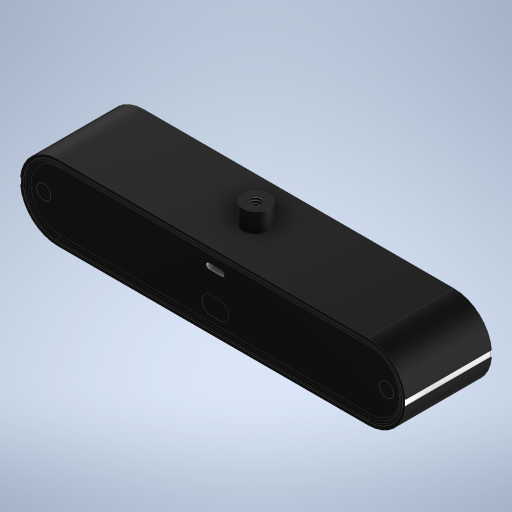
# Autodesk Inventor part: Astra
Saved by Autodesk Inventor 2024 (Build 280153000, 153)
## iProperties
Created: 2016-02-11
Part Number: Astra
Material: Generic
Document SubType Name: Modeling
Designer: John
Density: 1 g/cm^3
Appearance: Default
Author: John
Autodesk Inventor part; units mm, degrees
ref_plane "YZ Plane" through (0, 0, 0) normal (1, 0, 0) x (0, 1, 0)
ref_plane "XZ Plane" through (0, 0, 0) normal (0, 1, 0) x (-1, 0, 0)
sketch "Sketch1" plane through (0, 0, 0) normal (0, 1, 0) x (-1, 0, 0)
  line L0 (89.75, 0) -> (-89.75, 0) construction
  line L1 (72.2, 17.55) -> (-72.2, 17.55)
  line L2 (-72.2, -17.55) -> (72.2, -17.55)
  arc A0 (72.2, -17.55) -> (72.2, 17.55) centre (72.2, 0) ccw
  arc A1 (-72.2, 17.55) -> (-72.2, -17.55) centre (-72.2, 0) ccw
  point P0 (0, 0)
  point P1 (0, 0)
  dimension "d0" = 179.5
  dimension "d1" = 35.1
  constraints: 8 end point, 6 point on circle, 4 tangent, 2 centre point, 2 point on line, 1 coincident, 1 horizontal, 1 midpoint, 1 parallel
  measures "d0" distance of L0.start L0.end
  measures "d1" diameter of A1
extrude "Extrusion1" add sketch "Sketch1" along normal blind 40
sketch "Sketch2" plane through (0, 40, 0) normal (0, 1, 0) x (1, 0, 0)
  line L0 (-72.2, -17.55) -> (72.2, -17.55) projected
  arc A0 (72.2, -17.55) -> (72.2, 17.55) centre (72.2, 0) ccw projected
  line L1 (72.2, 17.55) -> (-72.2, 17.55) projected
  arc A1 (-72.2, 17.55) -> (-72.2, -17.55) centre (-72.2, 0) ccw projected
  line L2 (-72.2, 16.05) -> (72.2, 16.05)
  arc A2 (72.2, -16.05) -> (72.2, 16.05) centre (72.2, 0) ccw
  line L3 (72.2, -16.05) -> (-72.2, -16.05)
  arc A3 (-72.2, 16.05) -> (-72.2, -16.05) centre (-72.2, 0) ccw
  line L4 (-72.2, -14.55) -> (72.2, -14.55)
  arc A4 (72.2, -14.55) -> (72.2, 14.55) centre (72.2, 0) ccw
  line L5 (72.2, 14.55) -> (-72.2, 14.55)
  arc A5 (-72.2, 14.55) -> (-72.2, -14.55) centre (-72.2, 0) ccw
  point P0 (0, 0)
  dimension "d4" = 1.5
  dimension "d5" = 1.5
  constraints: 8 end point, 8 point on circle, 4 centre point, 6 other
  measures "d4" distance between parallel lines of L1 L2
  measures "d5" distance between parallel lines of L3 L4
extrude "Extrusion2" cut sketch "Sketch2" against normal blind 1 contours A5 L5 A4 L4
fillet "Fillet1" radius 1 8 edges at (-86.75, 39, 0) (0, 39, -14.55) (86.75, 39, 0) (0, 39, 14.55) (-86.75, 40, 0) (0, 40, -14.55) (86.75, 40, 0) (0, 40, 14.55)
sketch "Sketch3" plane through (0, 40, 0) normal (0, 1, 0) x (1, 0, 0)
  line L0 (-72.2, -17.55) -> (72.2, -17.55) projected
  arc A0 (72.2, -17.55) -> (72.2, 17.55) centre (72.2, 0) ccw projected
  line L1 (72.2, 17.55) -> (-72.2, 17.55) projected
  arc A1 (-72.2, 17.55) -> (-72.2, -17.55) centre (-72.2, 0) ccw projected
  arc A2 (-72.2, 15.2821) -> (-72.2, -15.2821) centre (-72.2, 0) ccw projected
  line L2 (72.2, 15.2821) -> (-72.2, 15.2821) projected
  arc A3 (72.2, -15.2821) -> (72.2, 15.2821) centre (72.2, 0) ccw projected
  line L3 (-72.2, -15.2821) -> (72.2, -15.2821) projected
  arc A4 (72.2, -15.95) -> (72.2, 15.95) centre (72.2, 0) ccw
  line L4 (72.2, 15.95) -> (-72.2, 15.95)
  arc A5 (-72.2, 15.95) -> (-72.2, -15.95) centre (-72.2, 0) ccw
  line L5 (-72.2, -15.95) -> (72.2, -15.95)
  line L6 (72.2, -16.05) -> (-72.2, -16.05)
  arc A6 (-72.2, 16.05) -> (-72.2, -16.05) centre (-72.2, 0) ccw
  line L7 (-72.2, 16.05) -> (72.2, 16.05)
  arc A7 (72.2, -16.05) -> (72.2, 16.05) centre (72.2, 0) ccw
  point P0 (0, 0)
  dimension "d12" = 1.5
  dimension "d13" = 0.1
  constraints: 8 end point, 8 point on circle, 4 centre point, 6 other
  measures "d12" distance between parallel lines of L0 L6
  measures "d13" distance between parallel lines of L5 L6
extrude "Extrusion3" cut sketch "Sketch3" against normal blind 1 contours L5 A5 L4 A4 | L6 A6 L7 A7
sketch "Sketch4" plane through (0, 0, 0) normal (0, -1, 0) x (1, 0, 0)
  line L0 (-72.2, 17.55) -> (72.2, 17.55) projected
  arc A0 (-72.2, 17.55) -> (-72.2, -17.55) centre (-72.2, 0) ccw projected
  line L1 (72.2, -17.55) -> (-72.2, -17.55) projected
  arc A1 (72.2, -17.55) -> (72.2, 17.55) centre (72.2, 0) ccw projected
  line L2 (72.2, 16.05) -> (-72.2, 16.05)
  arc A2 (-72.2, 16.05) -> (-72.2, -16.05) centre (-72.2, 0) ccw
  line L3 (-72.2, -16.05) -> (72.2, -16.05)
  arc A3 (72.2, -16.05) -> (72.2, 16.05) centre (72.2, 0) ccw
  line L4 (-72.2, 14.55) -> (72.2, 14.55)
  arc A4 (72.2, -14.55) -> (72.2, 14.55) centre (72.2, 0) ccw
  line L5 (72.2, -14.55) -> (-72.2, -14.55)
  arc A5 (-72.2, 14.55) -> (-72.2, -14.55) centre (-72.2, 0) ccw
  point P0 (0, 0)
  dimension "d14" = 1.5
  dimension "d15" = 1.5
  constraints: 8 end point, 8 point on circle, 4 centre point, 6 other
  measures "d14" distance between parallel lines of L0 L2
  measures "d15" distance between parallel lines of L2 L4
extrude "Extrusion4" cut sketch "Sketch4" against normal blind 1 contours L4 A4 L5 A5
fillet "Fillet2" radius 1 8 edges at (86.75, 1, 0) (0, 1, -14.55) (-86.75, 1, 0) (0, 1, 14.55) (86.75, 0, 0) (0, 0, -14.55) (-86.75, 0, 0) (0, 0, 14.55)
sketch "Sketch5" plane through (0, 0, 0) normal (0, -1, 0) x (1, 0, 0)
  line L0 (-72.2, 17.55) -> (72.2, 17.55) projected
  arc A0 (-72.2, 17.55) -> (-72.2, -17.55) centre (-72.2, 0) ccw projected
  line L1 (72.2, -17.55) -> (-72.2, -17.55) projected
  arc A1 (72.2, -17.55) -> (72.2, 17.55) centre (72.2, 0) ccw projected
  arc A2 (72.2, -15.2821) -> (72.2, 15.2821) centre (72.2, 0) ccw projected
  line L2 (-72.2, -15.2821) -> (72.2, -15.2821) projected
  arc A3 (-72.2, 15.2821) -> (-72.2, -15.2821) centre (-72.2, 0) ccw projected
  line L3 (72.2, 15.2821) -> (-72.2, 15.2821) projected
  line L4 (72.2, 16.05) -> (-72.2, 16.05)
  arc A4 (-72.2, 16.05) -> (-72.2, -16.05) centre (-72.2, 0) ccw
  line L5 (-72.2, -16.05) -> (72.2, -16.05)
  arc A5 (72.2, -16.05) -> (72.2, 16.05) centre (72.2, 0) ccw
  line L6 (-72.2, 16.15) -> (72.2, 16.15)
  arc A6 (72.2, -16.15) -> (72.2, 16.15) centre (72.2, 0) ccw
  line L7 (72.2, -16.15) -> (-72.2, -16.15)
  arc A7 (-72.2, 16.15) -> (-72.2, -16.15) centre (-72.2, 0) ccw
  point P0 (0, 0)
  dimension "d19" = 1.5
  dimension "d20" = 0.1
  constraints: 8 end point, 8 point on circle, 4 centre point, 6 other
  measures "d19" distance between parallel lines of L0 L4
  measures "d20" distance between parallel lines of L4 L6
extrude "Extrusion5" cut sketch "Sketch5" against normal blind 1 contours L6 A6 L7 A7
sketch "Sketch6" plane through (0, 39, 0) normal (0, 1, 0) x (1, 0, 0)
  line L0 (0, 0) -> (-60.5, 0) construction
  arc A0 (-61, 0.9108) -> (-61, -0.9108) centre (-60.5, 0) ccw construction
  arc A1 (-61.2406, 1.3491) -> (-61.2406, -1.3491) centre (-60.5, 0) ccw
  arc A2 (-60.7594, 0.4725) -> (-60.7594, -0.4725) centre (-60.5, 0) ccw
  arc A3 (-60.7594, 0.4725) -> (-61.2406, 1.3491) centre (-61, 0.9108) ccw
  arc A4 (-61.2406, -1.3491) -> (-60.7594, -0.4725) centre (-61, -0.9108) ccw
  line L1 (-60.5, 1) -> (-60.5, -1) construction
  dimension "d23" = 60.5
  dimension "d25" = 0.5
  dimension "d26" = 1
  dimension "d27" = 1
  dimension "d28" = 0
  constraints: 10 point on circle, 6 tangent, 5 centre point, 4 end point, 1 coincident, 1 horizontal, 1 vertical
  measures "d23" distance of L0.start L0.end
  measures "d25" radius of A3
  measures "d26" distance of L0.end L1.end
  measures "d27" distance of L0.end L1.start
  measures "d28" distance from line of L1 L0.end
extrude "mic" cut sketch "Sketch6" against normal blind 2
mirror "Mirror1" about plane through (0, 0, 0) normal (1, 0, 0) of "mic"
sketch "Sketch7" plane through (0, 39, 0) normal (0, 1, 0) x (1, 0, 0)
  circle A0 centre (-44, 0) radius 6.75
  circle A1 centre (5.5, 0) radius 6.75
  circle A2 centre (44, 0) radius 6.75
  line L0 (-50.75, 0) -> (-50.75, 30.3694) construction
  line L1 (50.0987, 2.8927) -> (50.0987, 29.071) construction
  line L2 (12.25, 0) -> (37.25, 0) construction
  line L3 (-50.75, 0) -> (50.75, 0) construction
  arc A3 (-72.2, 17.55) -> (-72.2, -17.55) centre (-72.2, 0) ccw construction
  arc A4 (72.2, -17.55) -> (72.2, 17.55) centre (72.2, 0) ccw construction
  line L4 (-89.75, 0) -> (-50.75, 0) construction
  line L5 (50.75, 0) -> (89.75, 0) construction
  point P0 (0, 0)
  dimension "d31" = 13.5
  dimension "d32" = 13.5
  dimension "d33" = 13.5
  dimension "d35" = 25
  dimension "d36" = 39
  dimension "d38" = 39
  constraints: 12 end point, 5 point on circle, 3 vertical, 2 collinear, 2 horizontal, 2 horizontal alignment, 2 point on line, 1 centre point, 4 other
  measures "d33" diameter of A2
  measures "d35" distance of L2.start L2.end
  measures "d36" distance of L4.start L0.start
  measures "d38" distance of L3.end L5.end
extrude "Extrusion7" cut sketch "Sketch7" against normal blind 1
chamfer "Chamfer1" distance 1 angle 45 3 edges at (37.25, 39, 0) (-1.25, 39, 0) (-50.75, 39, 0)
sketch "Sketch8" plane through (5.5, 38, 0) normal (0, 1, 0) x (1, 0, 0)
  circle A0 centre (0, 0) radius 6.75 projected
  circle A1 centre (38.5, 0) radius 6.75 projected
  circle A2 centre (-49.5, 0) radius 6.75 projected
  circle A3 centre (-49.5, 0) radius 5.75
  circle A4 centre (0, 0) radius 5.75
  circle A5 centre (38.5, 0) radius 5.75
  point P0 (-5.5, 0)
  dimension "d44" = 1
  dimension "d45" = 1
  dimension "d46" = 1
  constraints: 3 centre point
  measures "d44" radial gap between concentric circles of A2 A3
  measures "d45" radial gap between concentric circles of A0 A4
  measures "d46" radial gap between concentric circles of A1 A5
extrude "Extrusion8" cut sketch "Sketch8" against normal blind 0.5 contours A3 | A4 | A5
sketch "Sketch9" plane through (-44, 37.5, 0) normal (0, 1, 0) x (1, 0, 0)
  circle A0 centre (0, 0) radius 5.75 projected
  circle A1 centre (49.5, 0) radius 5.75 projected
  circle A2 centre (88, 0) radius 5.75 projected
  circle A3 centre (0, 0) radius 4.75
  circle A4 centre (49.5, 0) radius 4.75
  circle A5 centre (88, 0) radius 4.75
  point P0 (44, 0)
  dimension "d49" = 1
  dimension "d50" = 1
  dimension "d51" = 1
  constraints: 3 centre point
  measures "d49" radial gap between concentric circles of A0 A3
  measures "d50" radial gap between concentric circles of A1 A4
  measures "d51" radial gap between concentric circles of A2 A5
extrude "Extrusion9" cut sketch "Sketch9" against normal blind 0.5 contours A3 | A4 | A5
sketch "Sketch10" plane through (-44, 37, 0) normal (0, 1, 0) x (1, 0, 0)
  circle A0 centre (0, 0) radius 4.75 projected
  circle A1 centre (49.5, 0) radius 4.75 projected
  circle A2 centre (88, 0) radius 4.75 projected
  circle A3 centre (0, 0) radius 3.75
  circle A4 centre (49.5, 0) radius 3.75
  circle A5 centre (88, 0) radius 3.75
  point P0 (44, 0)
  dimension "d54" = 1
  dimension "d55" = 1
  dimension "d56" = 1
  constraints: 3 centre point
  measures "d54" radial gap between concentric circles of A0 A3
  measures "d55" radial gap between concentric circles of A1 A4
  measures "d56" radial gap between concentric circles of A2 A5
extrude "Extrusion10" cut sketch "Sketch10" against normal blind 0.5 contours A3 | A4 | A5
sketch "Sketch11" plane through (-44, 36.5, 0) normal (0, 1, 0) x (1, 0, 0)
  circle A0 centre (0, 0) radius 3.75 projected
  circle A1 centre (49.5, 0) radius 3.75 projected
  circle A2 centre (88, 0) radius 3.75 projected
  line L0 (-2, 2) -> (2, 2)
  line L1 (2, 2) -> (2, -2)
  line L2 (2, -2) -> (-2, -2)
  line L3 (-2, -2) -> (-2, 2)
  line L4 (-2, 2) -> (2, -2) construction
  line L5 (2, 2) -> (-2, -2) construction
  arc A3 (2, 2) -> (-2, 2) centre (0, 0) ccw
  arc A4 (-2, -2) -> (2, -2) centre (0, 0) ccw
  circle A5 centre (49.5, 0) radius 2
  circle A6 centre (88, 0) radius 2
  point P0 (44, 0)
  dimension "d59" = 4
  dimension "d60" = 4
  dimension "d61" = 4
  dimension "d62" = 4
  constraints: 12 end point, 4 centre point, 4 point on circle, 2 coincident, 2 concentric, 2 midpoint, 2 parallel, 1 horizontal, 1 perpendicular
  measures "d59" distance of L1.end L2.end
  measures "d60" distance of L0.end L1.end
  measures "d61" diameter of A5
  measures "d62" diameter of A6
extrude "Extrusion11" cut sketch "Sketch11" against normal blind 0.5 contours A3 L0 | L0 L1 L2 L3 | L2 A4 | A5 | A6
sketch "Sketch12" plane through (0, 39, 0) normal (0, 1, 0) x (1, 0, 0)
  circle A0 centre (-29.25, 5) radius 1.75
  circle A1 centre (-29.25, -5) radius 1.75
  line L0 (-29.25, 3.25) -> (-29.25, -3.25) construction
  line L1 (0, 0) -> (-55.288, 0) construction
  circle A2 centre (-44, 0) radius 7.75 projected
  point P0 (-36.25, 0)
  dimension "d65" = 3.5
  dimension "d66" = 3.5
  dimension "d67" = 6.5
  dimension "d68" = 3.25
  dimension "d69" = 7
  constraints: 4 end point, 2 vertical alignment, 1 horizontal, 1 horizontal alignment, 1 point on line, 1 vertical, 5 other
  measures "d67" distance of L0.start L0.end
  measures "d68" distance from line of L1 L0.start
  measures "d69" distance from line of L0 point (-36.25, 0)
extrude "Extrusion12" cut sketch "Sketch12" against normal blind 5 contours A0 | A1
chamfer "Chamfer2" distance 0.5 angle 45 2 edges at (-31, 39, -5) (-31, 39, 5)
sketch "Sketch13" plane through (-29.25, 34, -5) normal (0, 1, 0) x (1, 0, 0)
  circle A0 centre (0, 0) radius 1.75 projected
  circle A1 centre (0, -10) radius 1.75 projected
  circle A2 centre (0, -10) radius 1.55
  circle A3 centre (0, 0) radius 1.55
  point P0 (29.25, -5)
  dimension "d76" = 0.2
  dimension "d77" = 0.2
  constraints: 2 centre point
  measures "d76" radial gap between concentric circles of A1 A2
  measures "d77" radial gap between concentric circles of A0 A3
extrude "Extrusion13" add sketch "Sketch13" along normal blind 4 contours A2 | A3
fillet "Fillet3" radius 1 2 edges at (-30.8, 38, -5) (-30.8, 38, 5)
sketch "Sketch14" plane through (0, 1, 0) normal (0, -1, 0) x (1, 0, 0)
  circle A0 centre (79.75, 0) radius 3.375
  arc A1 (72.2, -17.55) -> (72.2, 17.55) centre (72.2, 0) ccw projected
  arc A2 (72.2, -17.55) -> (72.2, 17.55) centre (72.2, 0) ccw projected
  line L0 (89.75, 0) -> (89.75, -20.9344) construction
  circle A3 centre (79.75, 0) radius 3.275
  point P0 (0, 0)
  dimension "d81" = 6.75
  dimension "d82" = 10
  dimension "d83" = 0.1
  constraints: 2 centre point, 2 end point, 2 point on circle, 1 tangent, 1 vertical
  measures "d81" diameter of A0
  measures "d82" distance from line of A0.centre L0
  measures "d83" radial gap between concentric circles of A0 A3
extrude "Extrusion14" cut sketch "Sketch14" against normal blind 0.01
mirror "Mirror2" about plane through (0, 0, 0) normal (1, 0, 0) of "Extrusion14"
sketch "Sketch15" plane through (0, 1, 0) normal (0, -1, 0) x (1, 0, 0)
  line L0 (-6.25, -6.825) -> (6.25, -6.825) construction
  line L1 (-2.025, -11.05) -> (2.025, -11.05)
  line L2 (2.025, -2.6) -> (-2.025, -2.6)
  arc A0 (-2.025, -2.6) -> (-2.025, -11.05) centre (-2.025, -6.825) ccw
  arc A1 (2.025, -11.05) -> (2.025, -2.6) centre (2.025, -6.825) ccw
  line L3 (0, 0) -> (0, -6.825) construction
  line L4 (72.2, -17.55) -> (-72.2, -17.55) projected
  dimension "d86" = 12.5
  dimension "d87" = 8.45
  dimension "d88" = 6.5
  constraints: 10 end point, 6 point on circle, 4 tangent, 2 centre point, 2 point on line, 1 coincident, 1 horizontal, 1 midpoint, 1 parallel, 1 vertical
  measures "d86" distance of L0.start L0.end
  measures "d87" diameter of A1
  measures "d88" distance between parallel lines of L4 L1
extrude "Extrusion15" cut sketch "Sketch15" against normal blind 0.1
ref_plane "Work Plane2" through (0, -7, 0) normal (0, -1, 0) x (1, 0, 0)
sketch "Sketch19" plane through (0, -7, 0) normal (0, -1, 0) x (1, 0, 0)
  line L0 (2.025, -8.5) -> (-2.025, -8.5)
  arc A0 (2.025, -8.5) -> (2.025, -0.05) centre (2.025, -4.275) ccw
  line L1 (-2.025, -0.05) -> (2.025, -0.05)
  arc A1 (-2.025, -0.05) -> (-2.025, -8.5) centre (-2.025, -4.275) ccw
  circle A2 centre (0, -4.275) radius 2.25
  circle A3 centre (0, -4.275) radius 4.05
  line L2 (0, -6.525) -> (0, -8.325) construction
  line L3 (2.25, -4.275) -> (4.05, -4.275) construction
  line L4 (1.0482, -8.187) -> (0, -4.275) construction
  line L5 (0, -4.275) -> (3.912, -5.3232) construction
  line L6 (0.5823, -6.4483) -> (1.0482, -8.187)
  line L7 (2.1733, -4.8573) -> (3.912, -5.3232)
  point P0 (0, 0)
  dimension "d100" = 4.5
  dimension "d101" = 8.1
  dimension "d102" = 15
  dimension "d103" = 15
  constraints: 16 end point, 12 point on circle, 4 centre point, 2 collinear, 2 point on line, 1 coincident, 1 perpendicular, 1 vertical
  measures "d100" diameter of A2
  measures "d101" diameter of A3
  measures "d102" angle of L4 L2
  measures "d103" angle of L5 L3
extrude "Extrusion18" cut sketch "Sketch19" against normal blind 1 contours A2 L7 A3 L6 picked at (2.3707, -6.7566)
sketch "Sketch21" plane through (0, 40, 0) normal (0, 1, 0) x (1, 0, 0)
  arc A0 (72.2, -16.05) -> (72.2, 16.05) centre (72.2, 0) ccw projected
  line L0 (72.2, -16.05) -> (-72.2, -16.05) projected
  arc A1 (-72.2, 16.05) -> (-72.2, -16.05) centre (-72.2, 0) ccw projected
  line L1 (-72.2, 16.05) -> (72.2, 16.05) projected
  line L2 (-72.2, -17.55) -> (72.2, -17.55) projected
  arc A2 (72.2, -17.55) -> (72.2, 17.55) centre (72.2, 0) ccw projected
  line L3 (72.2, 17.55) -> (-72.2, 17.55) projected
  arc A3 (-72.2, 17.55) -> (-72.2, -17.55) centre (-72.2, 0) ccw projected
  line L4 (-89.25, 1.5) -> (-90.25, 1.5)
  line L5 (-90.25, 1.5) -> (-90.25, -1.5)
  line L6 (-90.25, -1.5) -> (-89.25, -1.5)
  line L7 (-89.25, -1.5) -> (-89.25, 1.5)
  arc A4 (-72.2, 17.55) -> (-72.2, -17.55) centre (-72.2, 0) ccw projected
  line L8 (-89.25, 1.5) -> (-90.25, -1.5) construction
  line L9 (-90.25, 1.5) -> (-89.25, -1.5) construction
  point P0 (0, 0)
  point P1 (-89.75, 0)
  dimension "d115" = 1
  dimension "d116" = 3
  constraints: 12 end point, 2 midpoint, 2 parallel, 2 point on circle, 1 horizontal, 1 perpendicular
  measures "d115" distance of L6.end L5.end
  measures "d116" distance of L5.end L4.end
extrude "Extrusion20" cut sketch "Sketch21" against normal up to next contours L6 L5 L4 A3 | A3 L4 L7 L6
mirror "Mirror3" about plane through (0, 0, 0) normal (1, 0, 0) of "Extrusion20"
sketch "Sketch24" plane through (-72.2, 0, 17.55) normal (0, 0, 1) x (1, 0, 0)
  line L0 (0, 0) -> (144.4, 0) projected
  line L1 (144.4, 0) -> (144.4, 40) projected
  line L2 (0, 40) -> (144.4, 40) projected
  line L3 (0, 0) -> (0, 40) projected
  circle A0 centre (72.2, 20) radius 6.1
  point P0 (72.2, 0)
  point P1 (72.2, 0)
  point P2 (144.4, 20)
  dimension "d122" = 12.2
  constraints: 2 midpoint, 1 centre point, 1 coincident, 1 horizontal alignment, 1 vertical alignment
  measures "d122" diameter of A0
extrude "Extrusion22" add sketch "Sketch24" along normal blind 9.1 contours A0
sketch "Sketch25" plane through (0, 20, 26.65) normal (0, 0, 1) x (1, 0, 0)
  circle A0 centre (0, 0) radius 6.1 projected
  point P0 (0, -20)
  constraints: 1 coincident
hole "Hole1" at (0, 20, 26.65) direction (0, 0, -1) diameter 4.9784 end through all thread size "1/4-20 UNC" class "2B" standard "ANSI Unified Screw Threads"
sketch "Sketch26" plane through (0, 1, 0) normal (0, -1, 0) x (1, 0, 0)
  arc A0 (2.025, -11.05) -> (2.025, -2.6) centre (2.025, -6.825) ccw projected
  line L0 (2.025, -11.05) -> (-2.025, -11.05) projected
  arc A1 (-2.025, -2.6) -> (-2.025, -11.05) centre (-2.025, -6.825) ccw projected
  line L1 (-2.025, -2.6) -> (2.025, -2.6) projected
  circle A2 centre (79.75, 0) radius 3.375 projected
  arc A3 (72.2, -13.55) -> (72.2, 13.55) centre (72.2, 0) ccw projected
  line L2 (-72.2, 13.55) -> (72.2, 13.55) projected
  arc A4 (-72.2, 13.55) -> (-72.2, -13.55) centre (-72.2, 0) ccw projected
  line L3 (72.2, -13.55) -> (-72.2, -13.55) projected
  circle A5 centre (-79.75, 0) radius 3.375 projected
  line L4 (-2.9, 8.55) -> (2.9, 8.55) construction
  line L5 (-2.9, 7.25) -> (2.9, 7.25)
  line L6 (2.9, 9.85) -> (-2.9, 9.85)
  arc A6 (-2.9, 9.85) -> (-2.9, 7.25) centre (-2.9, 8.55) ccw
  arc A7 (2.9, 7.25) -> (2.9, 9.85) centre (2.9, 8.55) ccw
  point P0 (0, 0)
  point P1 (0, 8.55)
  point P2 (-4.2, 8.55)
  point P3 (4.2, 8.55)
  point P4 (0, 13.55)
  dimension "d132" = 2.6
  dimension "d133" = 8.4
  dimension "d134" = 5
  constraints: 8 end point, 6 point on circle, 4 tangent, 2 centre point, 2 midpoint, 1 horizontal, 1 parallel, 1 vertical alignment
  measures "d132" diameter of A7
  measures "d133" distance of point (-4.2, 8.55) point (4.2, 8.55)
  measures "d134" distance from line of L2 point (0, 8.55)
extrude "Extrusion23" cut sketch "Sketch26" against normal blind 5 contours A6 L6 A7 L5
equation "\"d32\" = d31"
equation "\"d33\" = d31"
equation "\"d68\" = 0.5 * d67"
equation "\"d103\" = d102"
body "Solid1"
